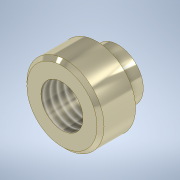
# Autodesk Inventor part: soldered nut
Saved by Autodesk Inventor 2022 (Build 260153000, 153)
## iProperties
Created: 2024-11-26
Part Number: soldered nut
Material: Типовые
Document SubType Name: Modeling
Designer: Andrey
Density: 1 g/cm^3
Appearance: Никель
Author: Andrey
Autodesk Inventor part; units mm, degrees
ref_plane "YZ Plane" through (0, 0, 0) normal (1, 0, 0) x (0, 1, 0)
ref_plane "XZ Plane" through (0, 0, 0) normal (0, 1, 0) x (-1, 0, 0)
ref_plane "XY Plane" through (0, 0, 0) normal (0, 0, 1) x (1, 0, 0)
sketch "Эскиз1" plane through (0, 0, 0) normal (0, 1, 0) x (-1, 0, 0)
  line L0 (0, 0) -> (2.75, 0)
  line L1 (2.75, 0) -> (2.75, 2.5)
  line L2 (2.75, 2.5) -> (-2.75, 2.5)
  line L3 (-2.75, 2.5) -> (-2.75, 0)
  line L4 (-2.75, 0) -> (2.75, 0)
  line L5 (0, 0) -> (1.8, 0)
  line L6 (1.8, 0) -> (1.8, -1.5)
  line L7 (1.8, -1.5) -> (-1.8, -1.5)
  line L8 (-1.8, -1.5) -> (-1.8, 0)
  line L9 (0, 2.5) -> (1.5, 2.5)
  line L10 (1.5, 2.5) -> (1.5, -1.5)
  line L11 (0, -1.5) -> (0, 2.5)
  dimension "d0" = 2.75
  dimension "d1" = 2.5
  dimension "d2" = 5.5
  dimension "d3" = 1.8
  dimension "d4" = 1.5
  dimension "d5" = 3.6
  dimension "d6" = 1.5
  constraints: 24 end point, 7 perpendicular, 5 point on line, 2 midpoint, 1 collinear, 1 horizontal
  measures "d0" distance of L0.start L0.end
  measures "d1" distance of L0.end L1.end
  measures "d2" distance of L1.end L2.end
  measures "d3" distance of L0.start L5.end
  measures "d4" distance of L5.end L6.end
  measures "d5" distance of L6.end L7.end
  measures "d6" distance of L9.start L9.end
revolve "Вращение1" add sketch "Эскиз1" angle 360 about axis through (0, 0, -1.5) along (0, 0, 1) contours L0 L10 L2 L1 | L6 L7 L10 L0
thread "Резьба1" size "M3x0.5" class "6H" standard "ANSI Metric M Profile" full length
chamfer "Фаска1" distance 0.25 angle 45 1 edges at (2.75, 0, 2.5)
